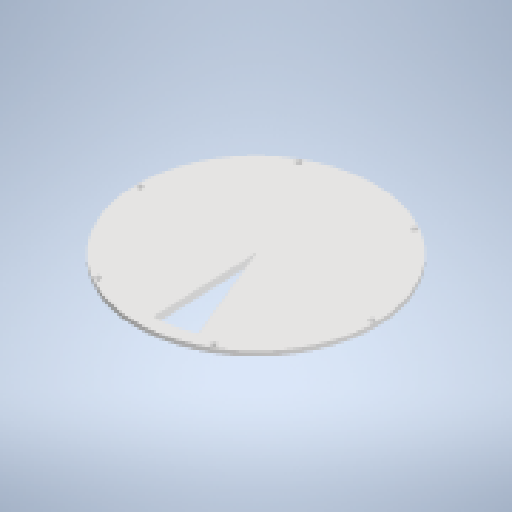
# Autodesk Inventor part: Bauteil3
Saved by Autodesk Inventor 2025 (Build 290162010, 162A)
## iProperties
Created: 2025-02-03
Part Number: Bauteil3
Material: Generisch
Document SubType Name: Modeling
Designer: Admin
Density: 1 g/cm^3
Appearance: Vorgabe
Author: Admin
Autodesk Inventor part; units mm, degrees
ref_plane "YZ Plane" through (0, 0, 0) normal (1, 0, 0) x (0, 1, 0)
ref_plane "XZ Plane" through (0, 0, 0) normal (0, 1, 0) x (-1, 0, 0)
ref_plane "XY Plane" through (0, 0, 0) normal (0, 0, 1) x (1, 0, 0)
sketch "Skizze1" plane through (0, 0, 0) normal (0, 0, 1) x (1, 0, 0)
  circle A0 centre (0, 0) radius 81 projected
  circle A1 centre (0, 0) radius 76 projected
  circle A2 centre (-78.5, 0) radius 0.4647 projected
  circle A3 centre (39.25, -67.983) radius 0.4647 projected
  circle A4 centre (78.5, 0) radius 0.4647 projected
  circle A5 centre (39.25, 67.983) radius 0.4647 projected
  circle A6 centre (-39.25, 67.983) radius 0.4647 projected
  circle A7 centre (-39.25, -67.983) radius 0.4647 projected
extrude "Extrusion1" add sketch "Skizze1" along normal blind 3 contours A0 | A1 | A2 | A3 | A4 | A5 | A6 | A7
sketch "Skizze2" plane through (0, 0, 3) normal (0, 0, 1) x (1, 0, 0)
  circle A0 centre (0, 0) radius 81 projected
  point P0 (-78.5, 0)
  point P1 (-39.25, -67.983)
  point P2 (39.25, -67.983)
  point P3 (78.5, 0)
  point P4 (39.25, 67.983)
  point P5 (-39.25, 67.983)
  dimension "d2" = 78.5
  dimension "d5" = 360
  constraints: 7 other
  measures "d2" distance of A0.centre point (-78.5, 0)
hole "Bohrung1" at (-78.5, 0, 3) at (-39.25, -67.983, 3) at (39.25, -67.983, 3) at (78.5, 0, 3) at (39.25, 67.983, 3) at (-39.25, 67.983, 3) direction (0, 0, -1) diameter 2.4 end through all countersink diameter 4.4 countersink angle 90 clearance for "Flachkopfmaschinenschraube" size "M2" standard "ANSI Metrisches M Profil"
sketch "Skizze3" plane through (0, 0, 3) normal (0, 0, 1) x (1, 0, 0)
  line L0 (2.1157, -9.7736) -> (25.0767, -65.2064) projected
  line L1 (4.1349, -69.7396) -> (2.1157, -9.7736) projected
  arc A0 (4.1349, -69.7396) -> (25.0767, -65.2064) centre (2.1157, -9.7736) ccw projected
  point P0 (0, 0)
extrude "Extrusion2" cut sketch "Skizze3" against normal through all
chamfer "Fasen1" distance 2 distance2 3 3 edges at (14.8098, -68.4154, 3) (3.1253, -39.7566, 3) (13.5962, -37.49, 3) measured on face at (2.6256, -39.7735, 3) measured on face at (14.0581, -37.2987, 3) measured on face at (14.9156, -68.9041, 3)
